Autodesk Inventor part; units mm, degrees
(part 4 of 4)
sketch "Эскиз10" plane through (23.5, 10.85, -93.6349) normal (0, 0, 1) x (1, 0, 0)
  arc A0 (0, 0) -> (-2.0546, 2.8471) centre (-3, 0) ccw projected
  line L0 (-2.0546, -10.85) -> (-2.0546, 2.8471) construction
  line L1 (0, -10.85) -> (-2.0546, -10.85) construction
  line L2 (0, -10.85) -> (0, 0) construction
  spline S0 degree 4 poles (-4.4081, 2.9941) (-4.3815, 2.997) (-4.3546, 2.999) (-4.3274, 3) (-4.3, 3) knots 0 0 0 0 0 1 1 1 1 1 projected
  line L3 (-4.4081, -1.0919) -> (-4.4081, 2.9941) construction
  line L4 (-3.5, -2) -> (-4.4081, -1.0919) projected
  line L5 (-3.5, -7) -> (-3.5, -2) construction
  line L6 (-4.4081, -7) -> (-3.5, -7) construction
  line L7 (-4.4081, -10.85) -> (-4.4081, -7) construction
  line L8 (-2.0546, -10.85) -> (-4.4081, -10.85) construction
  line L9 (-2.0546, -10.85) -> (-2.0546, 2.8471) construction
  spline S1 degree 6 poles (-3, 3) (-2.9139, 3) (-2.8267, 2.997) (-2.7386, 2.991) (-2.6499, 2.9817) (-2.5611, 2.9691) (-2.4019, 2.9407) (-2.3314, 2.926) (-2.2612, 2.9092) (-2.1915, 2.8904) (-2.1226, 2.8697) (-2.0546, 2.8471) knots 0 0 0 0 0 0 0 0.556009 0.556009 0.556009 0.556009 0.556009 1 1 1 1 1 1 1 projected
  line L10 (-4.3, 3) -> (-3, 3) projected
  arc A1 (-4.4081, 2.9941) -> (-5.3, 2) centre (-4.3, 2) ccw projected
  line L11 (-5.3, -0.2) -> (-5.3, 2) projected
  line L12 (-4.4081, -1.0919) -> (-5.3, -0.2) projected
  line L13 (-4.4081, -1.0919) -> (-4.4081, 2.9941) construction
  line L14 (-42.5919, -1.0919) -> (-42.5919, 2.9941) projected
  arc A2 (-41.7, 2) -> (-42.5919, 2.9941) centre (-42.7, 2) ccw projected
  line L15 (-42.5919, -1.0919) -> (-42.5919, 2.9941) projected
  line L16 (-41.7, -0.2) -> (-42.5919, -1.0919) projected
  line L17 (-41.7, -0.2) -> (-41.7, 2) projected
  spline S2 degree 7 poles (-42.7, 3) (-42.6843, 3) (-42.6687, 2.9997) (-42.6532, 2.9991) (-42.6378, 2.9983) (-42.6224, 2.9972) (-42.6071, 2.9958) (-42.5919, 2.9941) knots 0 0 0 0 0 0 0 0 1 1 1 1 1 1 1 1 projected
  line L18 (-44, 3) -> (-42.7, 3) projected
  spline S3 degree 5 poles (-44.9454, 2.8471) (-44.8643, 2.8741) (-44.782, 2.8982) (-44.6986, 2.9194) (-44.6145, 2.9376) (-44.4235, 2.9719) (-44.3163, 2.9862) (-44.2095, 2.9955) (-44.1039, 3) (-44, 3) knots 0 0 0 0 0 0 0.440959 0.440959 0.440959 0.440959 1 1 1 1 1 1 projected
  line L19 (-44.9454, -10.85) -> (-44.9454, 2.8471) construction
  line L20 (-42.5919, -10.85) -> (-44.9454, -10.85) construction
  line L21 (-42.5919, -10.85) -> (-42.5919, -7) construction
  line L22 (-43.5, -7) -> (-42.5919, -7) construction
  line L23 (-43.5, -7) -> (-43.5, -2) construction
  line L24 (-42.5919, -1.0919) -> (-43.5, -2) projected
  line L25 (-42.5919, -1.0919) -> (-42.5919, 2.9941) projected
  arc A3 (-44.9454, 2.8471) -> (-47, 0) centre (-44, 0) ccw projected
  line L26 (-47, -10.85) -> (-47, 0) construction
  line L27 (-44.9454, -10.85) -> (-47, -10.85) construction
  line L28 (-44.9454, -10.85) -> (-44.9454, 2.8471) construction
  line L29 (6.6851, -2.85) -> (-3.5, -2.85) construction
  line L30 (-3.0402, -2.85) -> (-3.5, -2.85) construction
  line L31 (0, -2.85) -> (-3.0402, -2.85) construction
  line L32 (0, -2.85) -> (1.5, -2.85) construction
  line L33 (1.5, -2.85) -> (3.522, -2.85) construction
  line L34 (3.522, -2.85) -> (6.6851, -2.85) construction
  line L35 (-43.5, -2.85) -> (-53.6851, -2.85) construction
  line L36 (-53.6851, -2.85) -> (-50.522, -2.85) construction
  line L37 (-50.522, -2.85) -> (-48.5, -2.85) construction
  line L38 (-48.5, -2.85) -> (-47, -2.85) construction
  line L39 (-43.9598, -2.85) -> (-47, -2.85) construction
  line L40 (-43.5, -2.85) -> (-43.9598, -2.85) construction
  line L41 (0, -10.85) -> (0, 0) projected
  line L42 (0, -2.85) -> (0, 0)
  line L43 (-3.5, -7) -> (-3.5, -2) projected
  line L44 (-3.5, -2.85) -> (-3.5, -2)
  line L45 (0, -2.85) -> (-3.5, -2.85)
  line L46 (-42.5919, -1.0919) -> (-43.5, -2) projected
  line L47 (-43.5, -2) -> (-43.5, -2.85)
  line L48 (-43.5, -7) -> (-43.5, -2) projected
  line L49 (-43.5, -2.85) -> (-47, -2.85)
  line L50 (-47, -10.85) -> (-47, 0) projected
  line L51 (-47, -2.85) -> (-47, 0)
  point P0 (-23.5, -10.85)
  point P1 (-44.9454, 2.8471)
  point P2 (-2.0546, 2.8471)
  constraints: 12 end point, 5 collinear, 1 perpendicular, 4 other
extrude "Выдавливание15" add sketch "Эскиз10" against normal blind 5.5
extrude "Выдавливание16" add sketch "Эскиз9" along normal up to surface (1.85 mm away) contours L103 A159 | A159 L103 A164 A165 A163 | A160 A161 L103 | L103 A162 A160 | A163 A165 A164 L106 L105 L104
fillet "Сопряжение3" radius 2 1 edges at (0, 2, -51)
sketch "Эскиз11" plane through (0, 0, 0) normal (0, -1, 0) x (1, 0, 0)
  circle A0 centre (0, -46) radius 1.6 projected
  circle A1 centre (24, -98.1071) radius 1.6 projected
  circle A2 centre (-24, -98.1071) radius 1.6 projected
  point P0 (0, 0)
extrude "Выдавливание17" cut sketch "Эскиз11" against normal up to surface (8 mm away)
